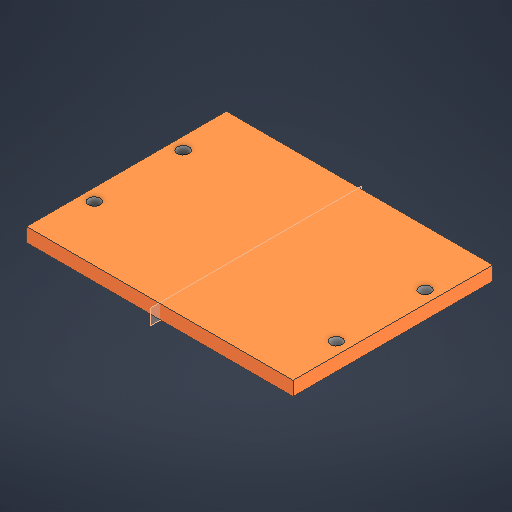
# Autodesk Inventor part: cooling plate
Saved by Autodesk Inventor 2026.2 (Build 302298000, 298)
## iProperties
Created: 2024-12-04
Part Number: cooling plate
Material: Generic
Document SubType Name: Modeling
Designer: cbast
Density: 1 g/cm^3
Appearance: Default
Author: cbast
Autodesk Inventor part; units mm, degrees
ref_plane "YZ Plane" through (0, 0, 0) normal (1, 0, 0) x (0, 1, 0)
ref_plane "XZ Plane" through (0, 0, 0) normal (0, 1, 0) x (-1, 0, 0)
ref_plane "XY Plane" through (0, 0, 0) normal (0, 0, 1) x (1, 0, 0)
sketch "Sketch1" plane through (0, 0, 0) normal (0, 1, 0) x (-1, 0, 0)
  line L0 (-76.2, 57.15) -> (76.2, 57.15)
  line L1 (76.2, 57.15) -> (76.2, -57.15)
  line L2 (76.2, -57.15) -> (-76.2, -57.15)
  line L3 (-76.2, -57.15) -> (-76.2, 57.15)
  line L4 (-76.2, 57.15) -> (76.2, -57.15) construction
  line L5 (76.2, 57.15) -> (-76.2, -57.15) construction
  point P0 (0, 0)
  dimension "d0" = 152.4
  dimension "d1" = 114.3
  constraints: 12 end point, 2 midpoint, 2 parallel, 1 horizontal, 1 perpendicular
  measures "d0" distance of L1.end L2.end
  measures "d1" distance of L0.end L1.end
extrude "Extrusion1" add sketch "Sketch1" along normal blind 8
sketch "Sketch10" plane through (0, 8, 0) normal (0, 1, 0) x (1, 0, 0)
  circle A0 centre (-69.2, 25.4) radius 3.365
  circle A1 centre (-69.2, -25.4) radius 3.365
  line L0 (-76.2, 57.15) -> (-76.2, -57.15) projected
  point P0 (0, 0)
  point P1 (-76.2, 0)
  dimension "d56" = 6.73
  dimension "d57" = 6.73
  dimension "d58" = 7
  dimension "d59" = 7
  dimension "d60" = 25.4
  dimension "d61" = 25.4
  constraints: 2 centre point, 1 midpoint
  measures "d56" diameter of A0
  measures "d57" diameter of A1
  measures "d58" distance from line of L0 A0.centre
  measures "d59" distance from line of L0 A1.centre
  measures "d60" vertical distance of point (-76.2, 0) A1.centre
  measures "d61" vertical distance of point (-76.2, 0) A0.centre
extrude "Extrusion10" cut sketch "Sketch10" against normal blind 10
ref_plane "Work Plane3" through (0, 0, 57.15) normal (1, 0, 0) x (0, 0, -1)
mirror "Mirror3" about plane through (0, 0, 57.15) normal (1, 0, 0) of "Extrusion10"
body "Solid1"
